Autodesk Fusion 360 part; units mm, degrees
(part 6 of 11)
  spline S88 degree 5 poles (-19.33, -28.8285) (-19.3279, -28.8303) (-19.3238, -28.8339) (-19.3174, -28.8391) (-19.3087, -28.8458) (-19.2974, -28.8537) (-19.286, -28.8614) (-19.2743, -28.8689) (-19.2626, -28.8762) (-19.2508, -28.8835) (-19.2389, -28.8907) (-19.227, -28.8979) (-19.215, -28.9049) (-19.2028, -28.9117) (-19.1905, -28.9185) (-19.1782, -28.925) (-19.1657, -28.9315) (-19.1531, -28.9379) (-19.1405, -28.9442) (-19.1278, -28.9504) (-19.1151, -28.9565) (-19.1022, -28.9625) (-19.0894, -28.9684) (-19.0764, -28.9743) (-19.0634, -28.98) (-19.0503, -28.9857) (-19.0371, -28.9913) (-19.0239, -28.9968) (-19.0106, -29.0022) (-18.9972, -29.0075) (-18.9838, -29.0128) (-18.9704, -29.0179) (-18.9569, -29.0231) (-18.9433, -29.0281) (-18.9297, -29.033) (-18.916, -29.0379) (-18.9023, -29.0427) (-18.8885, -29.0474) (-18.8746, -29.0521) (-18.8608, -29.0566) (-18.8468, -29.0612) (-18.8328, -29.0656) (-18.8188, -29.07) (-18.8047, -29.0742) (-18.7906, -29.0785) (-18.7764, -29.0826) (-18.7622, -29.0867) (-18.7479, -29.0907) (-18.7336, -29.0947) (-18.7193, -29.0985) (-18.7049, -29.1024) (-18.6905, -29.1061) (-18.676, -29.1098) (-18.6614, -29.1134) (-18.6469, -29.1169) (-18.6323, -29.1204) (-18.6176, -29.1238) (-18.6029, -29.1272) (-18.5882, -29.1304) (-18.5734, -29.1337) (-18.5586, -29.1368) (-18.5438, -29.1399) (-18.5289, -29.1429) (-18.514, -29.1459) (-18.499, -29.1488) (-18.484, -29.1516) (-18.469, -29.1544) (-18.4539, -29.1571) (-18.4388, -29.1597) (-18.4237, -29.1623) (-18.4085, -29.1648) (-18.3964, -29.1667) (-18.3872, -29.1682) (-18.3811, -29.1691) (-18.3781, -29.1696) knots 0 0 0 0 0 0 0.01428571 0.02857143 0.04285714 0.05714286 0.07142857 0.08571429 0.1 0.11428571 0.12857143 0.14285714 0.15714286 0.17142857 0.18571429 0.2 0.21428571 0.22857143 0.24285714 0.25714286 0.27142857 0.28571429 0.3 0.31428571 0.32857143 0.34285714 0.35714286 0.37142857 0.38571429 0.4 0.41428571 0.42857143 0.44285714 0.45714286 0.47142857 0.48571429 0.5 0.51428571 0.52857143 0.54285714 0.55714286 0.57142857 0.58571429 0.6 0.61428571 0.62857143 0.64285714 0.65714286 0.67142857 0.68571429 0.7 0.71428571 0.72857143 0.74285714 0.75714286 0.77142857 0.78571429 0.8 0.81428571 0.82857143 0.84285714 0.85714286 0.87142857 0.88571429 0.9 0.91428571 0.92857143 0.94285714 0.95714286 0.97142857 0.98571429 1 1 1 1 1 1 construction
  arc A179 (-18.3781, -29.1696) -> (-18.141, -28.8555) centre (-23.9648, -24.7074) ccw construction
  spline S89 degree 5 poles (-18.141, -28.8555) (-18.1423, -28.8527) (-18.1449, -28.8471) (-18.1488, -28.8387) (-18.154, -28.8275) (-18.1606, -28.8136) (-18.1672, -28.7998) (-18.1739, -28.786) (-18.1807, -28.7722) (-18.1874, -28.7585) (-18.1943, -28.7449) (-18.2012, -28.7313) (-18.2081, -28.7178) (-18.2151, -28.7043) (-18.2221, -28.6909) (-18.2292, -28.6775) (-18.2364, -28.6642) (-18.2435, -28.6509) (-18.2508, -28.6377) (-18.2581, -28.6245) (-18.2654, -28.6114) (-18.2728, -28.5984) (-18.2803, -28.5854) (-18.2878, -28.5725) (-18.2954, -28.5597) (-18.303, -28.5469) (-18.3107, -28.5341) (-18.3184, -28.5214) (-18.3261, -28.5088) (-18.334, -28.4963) (-18.3419, -28.4838) (-18.3498, -28.4714) (-18.3578, -28.459) (-18.3658, -28.4467) (-18.3739, -28.4345) (-18.3821, -28.4223) (-18.3903, -28.4102) (-18.3986, -28.3982) (-18.4069, -28.3862) (-18.4153, -28.3743) (-18.4237, -28.3625) (-18.4322, -28.3508) (-18.4408, -28.3391) (-18.4494, -28.3275) (-18.4581, -28.316) (-18.4668, -28.3046) (-18.4756, -28.2932) (-18.4844, -28.2819) (-18.4933, -28.2707) (-18.5023, -28.2595) (-18.5114, -28.2485) (-18.5205, -28.2376) (-18.5296, -28.2267) (-18.5389, -28.2159) (-18.5482, -28.2053) (-18.5576, -28.1947) (-18.567, -28.1842) (-18.5765, -28.1737) (-18.5861, -28.1634) (-18.5957, -28.1532) (-18.6054, -28.1431) (-18.6153, -28.1332) (-18.6252, -28.1234) (-18.6353, -28.1137) (-18.6454, -28.1042) (-18.6556, -28.0947) (-18.6658, -28.0854) (-18.6761, -28.0761) (-18.6865, -28.067) (-18.697, -28.0581) (-18.7077, -28.0494) (-18.7166, -28.0429) (-18.7233, -28.0382) (-18.7279, -28.0352) (-18.7303, -28.0337) knots -1 -1 -1 -1 -1 -1 -0.98571429 -0.97142857 -0.95714286 -0.94285714 -0.92857143 -0.91428571 -0.9 -0.88571429 -0.87142857 -0.85714286 -0.84285714 -0.82857143 -0.81428571 -0.8 -0.78571429 -0.77142857 -0.75714286 -0.74285714 -0.72857143 -0.71428571 -0.7 -0.68571429 -0.67142857 -0.65714286 -0.64285714 -0.62857143 -0.61428571 -0.6 -0.58571429 -0.57142857 -0.55714286 -0.54285714 -0.52857143 -0.51428571 -0.5 -0.48571429 -0.47142857 -0.45714286 -0.44285714 -0.42857143 -0.41428571 -0.4 -0.38571429 -0.37142857 -0.35714286 -0.34285714 -0.32857143 -0.31428571 -0.3 -0.28571429 -0.27142857 -0.25714286 -0.24285714 -0.22857143 -0.21428571 -0.2 -0.18571429 -0.17142857 -0.15714286 -0.14285714 -0.12857143 -0.11428571 -0.1 -0.08571429 -0.07142857 -0.05714286 -0.04285714 -0.02857143 -0.01428571 0 0 0 0 0 0 construction
  line L95 (-18.7303, -28.0337) -> (-18.788, -27.9968) construction
  arc A180 (-18.8697, -27.6608) -> (-18.788, -27.9968) centre (-18.6534, -27.7862) ccw construction
  arc A181 (-18.8697, -27.6608) -> (-18.8128, -27.5605) centre (-23.9648, -24.7074) ccw construction
  arc A182 (-18.4826, -27.4579) -> (-18.8128, -27.5605) centre (-18.5941, -27.6816) ccw construction
  line L96 (-18.4826, -27.4579) -> (-18.4213, -27.4885) construction
  spline S90 degree 5 poles (-18.4213, -27.4885) (-18.4188, -27.4897) (-18.4139, -27.4921) (-18.4064, -27.4955) (-18.3962, -27.4997) (-18.3833, -27.5045) (-18.3703, -27.5089) (-18.3571, -27.5131) (-18.3438, -27.5172) (-18.3306, -27.5211) (-18.3172, -27.5251) (-18.3039, -27.5288) (-18.2904, -27.5325) (-18.2769, -27.536) (-18.2633, -27.5393) (-18.2496, -27.5425) (-18.2359, -27.5455) (-18.2221, -27.5484) (-18.2083, -27.5512) (-18.1945, -27.5539) (-18.1806, -27.5565) (-18.1666, -27.559) (-18.1526, -27.5614) (-18.1386, -27.5637) (-18.1245, -27.5659) (-18.1104, -27.5679) (-18.0963, -27.5699) (-18.0821, -27.5718) (-18.0678, -27.5736) (-18.0536, -27.5753) (-18.0392, -27.5769) (-18.0249, -27.5784) (-18.0105, -27.5799) (-17.9961, -27.5812) (-17.9817, -27.5825) (-17.9672, -27.5836) (-17.9527, -27.5847) (-17.9382, -27.5857) (-17.9236, -27.5866) (-17.909, -27.5874) (-17.8944, -27.5882) (-17.8797, -27.5888) (-17.865, -27.5894) (-17.8503, -27.5899) (-17.8356, -27.5904) (-17.8208, -27.5907) (-17.806, -27.591) (-17.7912, -27.5912) (-17.7764, -27.5913) (-17.7615, -27.5913) (-17.7466, -27.5912) (-17.7317, -27.5911) (-17.7168, -27.5909) (-17.7018, -27.5907) (-17.6868, -27.5903) (-17.6718, -27.5899) (-17.6568, -27.5894) (-17.6417, -27.5888) (-17.6266, -27.5882) (-17.6115, -27.5875) (-17.5964, -27.5867) (-17.5813, -27.5858) (-17.5661, -27.5849) (-17.551, -27.5839) (-17.5358, -27.5828) (-17.5205, -27.5816) (-17.5053, -27.5804) (-17.4901, -27.5791) (-17.4748, -27.5778) (-17.4595, -27.5763) (-17.4442, -27.5748) (-17.4319, -27.5736) (-17.4227, -27.5726) (-17.4166, -27.5719) (-17.4135, -27.5716) knots 0 0 0 0 0 0 0.01428571 0.02857143 0.04285714 0.05714286 0.07142857 0.08571429 0.1 0.11428571 0.12857143 0.14285714 0.15714286 0.17142857 0.18571429 0.2 0.21428571 0.22857143 0.24285714 0.25714286 0.27142857 0.28571429 0.3 0.31428571 0.32857143 0.34285714 0.35714286 0.37142857 0.38571429 0.4 0.41428571 0.42857143 0.44285714 0.45714286 0.47142857 0.48571429 0.5 0.51428571 0.52857143 0.54285714 0.55714286 0.57142857 0.58571429 0.6 0.61428571 0.62857143 0.64285714 0.65714286 0.67142857 0.68571429 0.7 0.71428571 0.72857143 0.74285714 0.75714286 0.77142857 0.78571429 0.8 0.81428571 0.82857143 0.84285714 0.85714286 0.87142857 0.88571429 0.9 0.91428571 0.92857143 0.94285714 0.95714286 0.97142857 0.98571429 1 1 1 1 1 1 construction
  arc A183 (-17.4135, -27.5716) -> (-17.2659, -27.2069) centre (-23.9648, -24.7074) ccw construction
  spline S91 degree 5 poles (-17.2659, -27.2069) (-17.2678, -27.2045) (-17.2718, -27.1997) (-17.2777, -27.1926) (-17.2857, -27.1832) (-17.2956, -27.1715) (-17.3056, -27.1598) (-17.3156, -27.1482) (-17.3257, -27.1367) (-17.3358, -27.1252) (-17.3459, -27.1138) (-17.3561, -27.1025) (-17.3663, -27.0912) (-17.3765, -27.08) (-17.3868, -27.0688) (-17.3971, -27.0577) (-17.4075, -27.0467) (-17.4178, -27.0358) (-17.4283, -27.0249) (-17.4387, -27.0141) (-17.4492, -27.0033) (-17.4597, -26.9927) (-17.4703, -26.982) (-17.4809, -26.9715) (-17.4915, -26.9611) (-17.5022, -26.9507) (-17.5129, -26.9403) (-17.5236, -26.9301) (-17.5344, -26.9199) (-17.5452, -26.9098) (-17.5561, -26.8998) (-17.5669, -26.8898) (-17.5779, -26.88) (-17.5888, -26.8702) (-17.5998, -26.8605) (-17.6108, -26.8508) (-17.6219, -26.8413) (-17.633, -26.8318) (-17.6441, -26.8224) (-17.6553, -26.8131) (-17.6665, -26.8038) (-17.6778, -26.7947) (-17.689, -26.7856) (-17.7004, -26.7767) (-17.7117, -26.7678) (-17.7231, -26.759) (-17.7345, -26.7503) (-17.746, -26.7417) (-17.7575, -26.7332) (-17.7691, -26.7247) (-17.7807, -26.7164) (-17.7923, -26.7082) (-17.804, -26.7001) (-17.8157, -26.6921) (-17.8274, -26.6842) (-17.8392, -26.6764) (-17.8511, -26.6687) (-17.863, -26.6611) (-17.8749, -26.6536) (-17.8868, -26.6462) (-17.8988, -26.6389) (-17.9109, -26.6319) (-17.923, -26.625) (-17.9352, -26.6183) (-17.9475, -26.6117) (-17.9598, -26.6052) (-17.9721, -26.5988) (-17.9844, -26.5926) (-17.9968, -26.5864) (-18.0093, -26.5805) (-18.0219, -26.5749) (-18.0321, -26.5709) (-18.0399, -26.5681) (-18.0451, -26.5664) (-18.0477, -26.5656) knots -1 -1 -1 -1 -1 -1 -0.98571429 -0.97142857 -0.95714286 -0.94285714 -0.92857143 -0.91428571 -0.9 -0.88571429 -0.87142857 -0.85714286 -0.84285714 -0.82857143 -0.81428571 -0.8 -0.78571429 -0.77142857 -0.75714286 -0.74285714 -0.72857143 -0.71428571 -0.7 -0.68571429 -0.67142857 -0.65714286 -0.64285714 -0.62857143 -0.61428571 -0.6 -0.58571429 -0.57142857 -0.55714286 -0.54285714 -0.52857143 -0.51428571 -0.5 -0.48571429 -0.47142857 -0.45714286 -0.44285714 -0.42857143 -0.41428571 -0.4 -0.38571429 -0.37142857 -0.35714286 -0.34285714 -0.32857143 -0.31428571 -0.3 -0.28571429 -0.27142857 -0.25714286 -0.24285714 -0.22857143 -0.21428571 -0.2 -0.18571429 -0.17142857 -0.15714286 -0.14285714 -0.12857143 -0.11428571 -0.1 -0.08571429 -0.07142857 -0.05714286 -0.04285714 -0.02857143 -0.01428571 0 0 0 0 0 0 construction
  line L97 (-18.0477, -26.5656) -> (-18.113, -26.5449) construction
  arc A184 (-18.2789, -26.2414) -> (-18.113, -26.5449) centre (-18.0375, -26.3066) ccw construction
  arc A185 (-18.2789, -26.2414) -> (-18.2499, -26.1299) centre (-23.9648, -24.7074) ccw construction
  arc A186 (-17.9575, -25.9453) -> (-18.2499, -26.1299) centre (-18.0073, -26.1903) ccw construction
  line L98 (-17.9575, -25.9453) -> (-17.8904, -25.9589) construction
  spline S92 degree 5 poles (-17.8904, -25.9589) (-17.8877, -25.9595) (-17.8823, -25.9605) (-17.8742, -25.9619) (-17.8633, -25.9633) (-17.8496, -25.9646) (-17.8358, -25.9655) (-17.822, -25.9661) (-17.8082, -25.9666) (-17.7943, -25.967) (-17.7804, -25.9674) (-17.7665, -25.9676) (-17.7526, -25.9676) (-17.7386, -25.9675) (-17.7246, -25.9672) (-17.7106, -25.9667) (-17.6966, -25.966) (-17.6825, -25.9653) (-17.6685, -25.9644) (-17.6544, -25.9634) (-17.6403, -25.9623) (-17.6261, -25.9612) (-17.612, -25.9599) (-17.5979, -25.9584) (-17.5837, -25.9569) (-17.5695, -25.9553) (-17.5553, -25.9535) (-17.5411, -25.9516) (-17.5269, -25.9497) (-17.5127, -25.9476) (-17.4985, -25.9455) (-17.4842, -25.9433) (-17.47, -25.9409) (-17.4557, -25.9385) (-17.4414, -25.936) (-17.4272, -25.9333) (-17.4129, -25.9306) (-17.3986, -25.9278) (-17.3843, -25.9249) (-17.3699, -25.922) (-17.3556, -25.9189) (-17.3413, -25.9157) (-17.327, -25.9125) (-17.3126, -25.9092) (-17.2983, -25.9058) (-17.2839, -25.9023) (-17.2696, -25.8987) (-17.2552, -25.8951) (-17.2408, -25.8913) (-17.2265, -25.8875) (-17.2121, -25.8836) (-17.1977, -25.8796) (-17.1833, -25.8756) (-17.169, -25.8714) (-17.1546, -25.8672) (-17.1402, -25.8629) (-17.1258, -25.8586) (-17.1114, -25.8541) (-17.097, -25.8496) (-17.0826, -25.845) (-17.0682, -25.8403) (-17.0538, -25.8356) (-17.0394, -25.8307) (-17.025, -25.8258) (-17.0106, -25.8209) (-16.9962, -25.8158) (-16.9818, -25.8107) (-16.9674, -25.8055) (-16.953, -25.8002) (-16.9386, -25.7949) (-16.9242, -25.7895) (-16.9127, -25.7851) (-16.9041, -25.7818) (-16.8983, -25.7795) (-16.8954, -25.7784) knots 0 0 0 0 0 0 0.01428571 0.02857143 0.04285714 0.05714286 0.07142857 0.08571429 0.1 0.11428571 0.12857143 0.14285714 0.15714286 0.17142857 0.18571429 0.2 0.21428571 0.22857143 0.24285714 0.25714286 0.27142857 0.28571429 0.3 0.31428571 0.32857143 0.34285714 0.35714286 0.37142857 0.38571429 0.4 0.41428571 0.42857143 0.44285714 0.45714286 0.47142857 0.48571429 0.5 0.51428571 0.52857143 0.54285714 0.55714286 0.57142857 0.58571429 0.6 0.61428571 0.62857143 0.64285714 0.65714286 0.67142857 0.68571429 0.7 0.71428571 0.72857143 0.74285714 0.75714286 0.77142857 0.78571429 0.8 0.81428571 0.82857143 0.84285714 0.85714286 0.87142857 0.88571429 0.9 0.91428571 0.92857143 0.94285714 0.95714286 0.97142857 0.98571429 1 1 1 1 1 1 construction
  arc A187 (-16.8954, -25.7784) -> (-16.8472, -25.3879) centre (-23.9648, -24.7074) ccw construction
  spline S93 degree 5 poles (-16.8472, -25.3879) (-16.8497, -25.3861) (-16.8548, -25.3825) (-16.8624, -25.3772) (-16.8725, -25.3702) (-16.8851, -25.3614) (-16.8978, -25.3527) (-16.9105, -25.3441) (-16.9232, -25.3356) (-16.9359, -25.3271) (-16.9486, -25.3187) (-16.9614, -25.3104) (-16.9742, -25.3021) (-16.9869, -25.294) (-16.9998, -25.2858) (-17.0126, -25.2778) (-17.0254, -25.2698) (-17.0383, -25.262) (-17.0512, -25.2541) (-17.0641, -25.2464) (-17.077, -25.2387) (-17.0899, -25.2312) (-17.1029, -25.2236) (-17.1158, -25.2162) (-17.1288, -25.2089) (-17.1418, -25.2016) (-17.1548, -25.1944) (-17.1678, -25.1873) (-17.1809, -25.1802) (-17.1939, -25.1733) (-17.207, -25.1664) (-17.2201, -25.1596) (-17.2332, -25.1529) (-17.2463, -25.1463) (-17.2594, -25.1397) (-17.2726, -25.1333) (-17.2857, -25.1269) (-17.2989, -25.1206) (-17.3121, -25.1144) (-17.3253, -25.1083) (-17.3385, -25.1023) (-17.3517, -25.0964) (-17.365, -25.0906) (-17.3782, -25.0848) (-17.3915, -25.0792) (-17.4048, -25.0736) (-17.4181, -25.0682) (-17.4314, -25.0628) (-17.4447, -25.0576) (-17.4581, -25.0524) (-17.4714, -25.0474) (-17.4848, -25.0424) (-17.4982, -25.0376) (-17.5115, -25.0329) (-17.525, -25.0283) (-17.5384, -25.0239) (-17.5518, -25.0195) (-17.5652, -25.0152) (-17.5787, -25.0111) (-17.5921, -25.007) (-17.6056, -25.0032) (-17.6191, -24.9994) (-17.6326, -24.9959) (-17.6461, -24.9926) (-17.6597, -24.9894) (-17.6732, -24.9863) (-17.6868, -24.9834) (-17.7003, -24.9805) (-17.7139, -24.9778) (-17.7274, -24.9753) (-17.741, -24.9732) (-17.7519, -24.9719) (-17.7602, -24.9712) (-17.7656, -24.9709) (-17.7684, -24.9708) knots -1 -1 -1 -1 -1 -1 -0.98571429 -0.97142857 -0.95714286 -0.94285714 -0.92857143 -0.91428571 -0.9 -0.88571429 -0.87142857 -0.85714286 -0.84285714 -0.82857143 -0.81428571 -0.8 -0.78571429 -0.77142857 -0.75714286 -0.74285714 -0.72857143 -0.71428571 -0.7 -0.68571429 -0.67142857 -0.65714286 -0.64285714 -0.62857143 -0.61428571 -0.6 -0.58571429 -0.57142857 -0.55714286 -0.54285714 -0.52857143 -0.51428571 -0.5 -0.48571429 -0.47142857 -0.45714286 -0.44285714 -0.42857143 -0.41428571 -0.4 -0.38571429 -0.37142857 -0.35714286 -0.34285714 -0.32857143 -0.31428571 -0.3 -0.28571429 -0.27142857 -0.25714286 -0.24285714 -0.22857143 -0.21428571 -0.2 -0.18571429 -0.17142857 -0.15714286 -0.14285714 -0.12857143 -0.11428571 -0.1 -0.08571429 -0.07142857 -0.05714286 -0.04285714 -0.02857143 -0.01428571 0 0 0 0 0 0 construction
  line L99 (-17.7684, -24.9708) -> (-17.8368, -24.9677) construction
  arc A188 (-18.0756, -24.7176) -> (-17.8368, -24.9677) centre (-17.8256, -24.718) ccw construction
  arc A189 (-18.0756, -24.7176) -> (-18.0765, -24.6023) centre (-23.9648, -24.7074) ccw construction
  arc A190 (-17.8418, -24.3483) -> (-18.0765, -24.6023) centre (-17.8265, -24.5979) ccw construction
  line L100 (-17.8418, -24.3483) -> (-17.7734, -24.3441) construction
  spline S94 degree 5 poles (-17.7734, -24.3441) (-17.7707, -24.344) (-17.7652, -24.3436) (-17.757, -24.3428) (-17.7461, -24.3413) (-17.7326, -24.339) (-17.719, -24.3363) (-17.7055, -24.3333) (-17.692, -24.3303) (-17.6785, -24.3271) (-17.665, -24.3238) (-17.6515, -24.3204) (-17.6381, -24.3168) (-17.6246, -24.3131) (-17.6112, -24.3092) (-17.5978, -24.3051) (-17.5844, -24.3008) (-17.571, -24.2965) (-17.5577, -24.292) (-17.5443, -24.2874) (-17.531, -24.2827) (-17.5176, -24.2779) (-17.5043, -24.273) (-17.491, -24.2679) (-17.4777, -24.2628) (-17.4645, -24.2575) (-17.4512, -24.2522) (-17.438, -24.2467) (-17.4248, -24.2411) (-17.4116, -24.2355) (-17.3984, -24.2297) (-17.3852, -24.2239) (-17.372, -24.2179) (-17.3589, -24.2119) (-17.3457, -24.2057) (-17.3326, -24.1995) (-17.3195, -24.1932) (-17.3064, -24.1868) (-17.2934, -24.1803) (-17.2803, -24.1737) (-17.2673, -24.167) (-17.2542, -24.1603) (-17.2412, -24.1534) (-17.2282, -24.1465) (-17.2153, -24.1395) (-17.2023, -24.1324) (-17.1894, -24.1253) (-17.1764, -24.118) (-17.1635, -24.1107) (-17.1506, -24.1033) (-17.1378, -24.0958) (-17.1249, -24.0882) (-17.1121, -24.0806) (-17.0992, -24.0729) (-17.0864, -24.0651) (-17.0737, -24.0572) (-17.0609, -24.0493) (-17.0481, -24.0413) (-17.0354, -24.0332) (-17.0227, -24.025) (-17.01, -24.0168) (-16.9973, -24.0084) (-16.9847, -24) (-16.972, -23.9916) (-16.9594, -23.9831) (-16.9468, -23.9745) (-16.9342, -23.9658) (-16.9216, -23.957) (-16.9091, -23.9482) (-16.8966, -23.9393) (-16.8841, -23.9304) (-16.8741, -23.9232) (-16.8666, -23.9177) (-16.8616, -23.9141) (-16.8591, -23.9123) knots 0 0 0 0 0 0 0.01428571 0.02857143 0.04285714 0.05714286 0.07142857 0.08571429 0.1 0.11428571 0.12857143 0.14285714 0.15714286 0.17142857 0.18571429 0.2 0.21428571 0.22857143 0.24285714 0.25714286 0.27142857 0.28571429 0.3 0.31428571 0.32857143 0.34285714 0.35714286 0.37142857 0.38571429 0.4 0.41428571 0.42857143 0.44285714 0.45714286 0.47142857 0.48571429 0.5 0.51428571 0.52857143 0.54285714 0.55714286 0.57142857 0.58571429 0.6 0.61428571 0.62857143 0.64285714 0.65714286 0.67142857 0.68571429 0.7 0.71428571 0.72857143 0.74285714 0.75714286 0.77142857 0.78571429 0.8 0.81428571 0.82857143 0.84285714 0.85714286 0.87142857 0.88571429 0.9 0.91428571 0.92857143 0.94285714 0.95714286 0.97142857 0.98571429 1 1 1 1 1 1 construction
  arc A191 (-16.8591, -23.9123) -> (-16.9136, -23.5225) centre (-23.9648, -24.7074) ccw construction
  spline S95 degree 5 poles (-16.9136, -23.5225) (-16.9165, -23.5215) (-16.9223, -23.5193) (-16.931, -23.5162) (-16.9426, -23.512) (-16.9571, -23.5068) (-16.9715, -23.5017) (-16.986, -23.4966) (-17.0005, -23.4917) (-17.015, -23.4868) (-17.0295, -23.482) (-17.0439, -23.4772) (-17.0584, -23.4726) (-17.0729, -23.468) (-17.0874, -23.4635) (-17.1018, -23.459) (-17.1163, -23.4546) (-17.1308, -23.4504) (-17.1452, -23.4461) (-17.1597, -23.442) (-17.1742, -23.4379) (-17.1886, -23.434) (-17.2031, -23.4301) (-17.2175, -23.4262) (-17.2319, -23.4225) (-17.2464, -23.4188) (-17.2608, -23.4152) (-17.2752, -23.4117) (-17.2896, -23.4083) (-17.3041, -23.405) (-17.3185, -23.4017) (-17.3329, -23.3985) (-17.3472, -23.3955) (-17.3616, -23.3924) (-17.376, -23.3895) (-17.3904, -23.3867) (-17.4047, -23.3839) (-17.4191, -23.3813) (-17.4334, -23.3787) (-17.4478, -23.3762) (-17.4621, -23.3738) (-17.4764, -23.3715) (-17.4907, -23.3693) (-17.505, -23.3672) (-17.5193, -23.3652) (-17.5335, -23.3633) (-17.5478, -23.3615) (-17.562, -23.3598) (-17.5763, -23.3581) (-17.5905, -23.3566) (-17.6047, -23.3552) (-17.6189, -23.3539) (-17.633, -23.3527) (-17.6472, -23.3516) (-17.6613, -23.3507) (-17.6754, -23.3498) (-17.6895, -23.3491) (-17.7036, -23.3484) (-17.7177, -23.3479) (-17.7317, -23.3475) (-17.7457, -23.3472) (-17.7597, -23.3471) (-17.7737, -23.3472) (-17.7876, -23.3475) (-17.8015, -23.3479) (-17.8154, -23.3485) (-17.8292, -23.3491) (-17.8431, -23.3498) (-17.8569, -23.3507) (-17.8706, -23.3518) (-17.8843, -23.3533) (-17.8952, -23.3549) (-17.9033, -23.3564) (-17.9087, -23.3575) (-17.9114, -23.3581) knots -1 -1 -1 -1 -1 -1 -0.98571429 -0.97142857 -0.95714286 -0.94285714 -0.92857143 -0.91428571 -0.9 -0.88571429 -0.87142857 -0.85714286 -0.84285714 -0.82857143 -0.81428571 -0.8 -0.78571429 -0.77142857 -0.75714286 -0.74285714 -0.72857143 -0.71428571 -0.7 -0.68571429 -0.67142857 -0.65714286 -0.64285714 -0.62857143 -0.61428571 -0.6 -0.58571429 -0.57142857 -0.55714286 -0.54285714 -0.52857143 -0.51428571 -0.5 -0.48571429 -0.47142857 -0.45714286 -0.44285714 -0.42857143 -0.41428571 -0.4 -0.38571429 -0.37142857 -0.35714286 -0.34285714 -0.32857143 -0.31428571 -0.3 -0.28571429 -0.27142857 -0.25714286 -0.24285714 -0.22857143 -0.21428571 -0.2 -0.18571429 -0.17142857 -0.15714286 -0.14285714 -0.12857143 -0.11428571 -0.1 -0.08571429 -0.07142857 -0.05714286 -0.04285714 -0.02857143 -0.01428571 0 0 0 0 0 0 construction
  line L101 (-17.9114, -23.3581) -> (-17.9782, -23.3728) construction
  arc A192 (-18.2736, -23.193) -> (-17.9782, -23.3728) centre (-18.032, -23.1287) ccw construction
  circle A193 centre (-23.9648, -24.7074) radius 1.25 construction
  circle A194 centre (-23.9648, -24.7074) radius 1.225 construction
  circle A195 centre (-11.6741, -19.5) radius 1.225 construction
  line L102 (-7.5589, -33.5042) -> (-9.5095, -28.9004) construction
  line L103 (-9.5095, -28.9004) -> (-5.8324, -16.7546) construction
  arc A196 (-5.8324, -16.7546) -> (-7.9044, -14.1813) centre (-7.7466, -16.1751) ccw construction
  line L104 (-7.9044, -14.1813) -> (-14.4255, -14.1704) construction
  arc A197 (-14.4255, -14.1704) -> (-16.9722, -14.6854) centre (-14.4364, -20.6704) ccw construction
  line L105 (-16.9722, -14.6854) -> (-23.7382, -17.5521) construction
  arc A198 (-23.7382, -17.5521) -> (-25.8797, -19.0234) centre (-21.2025, -23.537) ccw construction
  line L106 (-25.8797, -19.0234) -> (-30.4081, -23.7158) construction
  arc A199 (-30.4081, -23.7158) -> (-30.0007, -26.9945) centre (-29.0855, -25.2161) ccw construction
  line L107 (-30.0007, -26.9945) -> (-18.7172, -32.8016) construction
  line L108 (-18.7172, -32.8016) -> (-16.7666, -37.4054) construction
  line L109 (-16.7666, -37.4054) -> (-7.5589, -33.5042) construction
  line L110 (-20.3552, -16.1187) -> (-12.1627, -35.4548) construction
  line L111 (-32.6369, -35.6954) -> (-24.2895, -27.0745)
  line L112 (-24.2895, -27.0745) -> (-25.7264, -25.6832)
  line L113 (-25.7264, -25.6832) -> (-34.0738, -34.3042)
  line L114 (-34.0738, -34.3042) -> (-32.6369, -35.6954)
  point P0 (-3.7477, -19.9132)
  dimension "d196" = 12
  dimension "d197" = 2
  constraint horizontal L48
  constraint perpendicular L48 L49
  constraint parallel L48 L50
  constraint parallel L49 L51
  constraint coincident L52 P0
  constraint coincident L53 P0
  constraint midpoint L105 L110.start
  constraint midpoint L109 L110.end
  constraint symmetric L48.start L110 L111.start
  constraint symmetric L48.end L110 L111.end
  constraint symmetric L49.end L110 L112.end
  constraint symmetric L50.end L110 L113.end
  measures "d196" distance of L49.end L50.end
  measures "d197" distance of L48.end L49.end
extrude "Extrude1''" add sketch "Sketch21" along normal blind 2 separate body contours A89 L44 S44 A90 S45 L45 A91 A92 A93 L46 S46 L48 L50 L51 | A89 L44 S44 A90 S45 L45 A91 A92 A93 L46 S46 L48 L49 L50 makes body 4 in component "Component"
sketch "Sketch22" plane through (0, 0, 5.45) normal (0, 0, 1) x (-1, 0, 0)
  arc A0 (-17.5052, -18.6742) -> (-17.5202, -18.7885) centre (-11.6741, -19.5) ccw
  arc A1 (-17.7878, -19.0075) -> (-17.5202, -18.7885) centre (-17.7684, -18.7583) ccw
  line L0 (-17.7878, -19.0075) -> (-17.8561, -19.0022)
  spline S0 degree 5 poles (-17.8561, -19.0022) (-17.8588, -19.002) (-17.8643, -19.0016) (-17.8726, -19.0013) (-17.8835, -19.0012) (-17.8973, -19.0016) (-17.9111, -19.0024) (-17.9249, -19.0035) (-17.9387, -19.0046) (-17.9525, -19.0059) (-17.9663, -19.0073) (-17.9801, -19.0088) (-17.9939, -19.0105) (-18.0078, -19.0123) (-18.0216, -19.0143) (-18.0355, -19.0165) (-18.0493, -19.0189) (-18.0632, -19.0214) (-18.077, -19.024) (-18.0909, -19.0267) (-18.1048, -19.0295) (-18.1186, -19.0324) (-18.1325, -19.0354) (-18.1463, -19.0385) (-18.1602, -19.0418) (-18.1741, -19.0452) (-18.188, -19.0486) (-18.2018, -19.0522) (-18.2157, -19.0559) (-18.2295, -19.0597) (-18.2434, -19.0636) (-18.2573, -19.0675) (-18.2711, -19.0716) (-18.285, -19.0758) (-18.2989, -19.08) (-18.3127, -19.0844) (-18.3266, -19.0888) (-18.3404, -19.0933) (-18.3542, -19.098) (-18.3681, -19.1027) (-18.3819, -19.1075) (-18.3958, -19.1123) (-18.4096, -19.1173) (-18.4234, -19.1224) (-18.4372, -19.1275) (-18.4511, -19.1327) (-18.4649, -19.138) (-18.4787, -19.1434) (-18.4925, -19.1489) (-18.5063, -19.1544) (-18.52, -19.1601) (-18.5338, -19.1658) (-18.5476, -19.1716) (-18.5614, -19.1774) (-18.5751, -19.1834) (-18.5889, -19.1894) (-18.6026, -19.1955) (-18.6164, -19.2017) (-18.6301, -19.2079) (-18.6438, -19.2143) (-18.6575, -19.2207) (-18.6712, -19.2271) (-18.6849, -19.2337) (-18.6986, -19.2403) (-18.7123, -19.247) (-18.726, -19.2538) (-18.7397, -19.2606) (-18.7533, -19.2676) (-18.767, -19.2746) (-18.7806, -19.2816) (-18.7942, -19.2887) (-18.8051, -19.2945) (-18.8133, -19.2989) (-18.8187, -19.3018) (-18.8214, -19.3032) knots 0 0 0 0 0 0 0.01428571 0.02857143 0.04285714 0.05714286 0.07142857 0.08571429 0.1 0.11428571 0.12857143 0.14285714 0.15714286 0.17142857 0.18571429 0.2 0.21428571 0.22857143 0.24285714 0.25714286 0.27142857 0.28571429 0.3 0.31428571 0.32857143 0.34285714 0.35714286 0.37142857 0.38571429 0.4 0.41428571 0.42857143 0.44285714 0.45714286 0.47142857 0.48571429 0.5 0.51428571 0.52857143 0.54285714 0.55714286 0.57142857 0.58571429 0.6 0.61428571 0.62857143 0.64285714 0.65714286 0.67142857 0.68571429 0.7 0.71428571 0.72857143 0.74285714 0.75714286 0.77142857 0.78571429 0.8 0.81428571 0.82857143 0.84285714 0.85714286 0.87142857 0.88571429 0.9 0.91428571 0.92857143 0.94285714 0.95714286 0.97142857 0.98571429 1 1 1 1 1 1
  arc A2 (-18.8214, -19.3032) -> (-18.8214, -19.6968) centre (-11.6741, -19.5) ccw
  spline S1 degree 5 poles (-18.8214, -19.6968) (-18.8187, -19.6982) (-18.8133, -19.7011) (-18.8051, -19.7055) (-18.7942, -19.7113) (-18.7806, -19.7184) (-18.767, -19.7254) (-18.7533, -19.7324) (-18.7397, -19.7394) (-18.726, -19.7462) (-18.7123, -19.753) (-18.6986, -19.7597) (-18.6849, -19.7663) (-18.6712, -19.7729) (-18.6575, -19.7793) (-18.6438, -19.7857) (-18.6301, -19.7921) (-18.6164, -19.7983) (-18.6026, -19.8045) (-18.5889, -19.8106) (-18.5751, -19.8166) (-18.5614, -19.8226) (-18.5476, -19.8284) (-18.5338, -19.8342) (-18.52, -19.8399) (-18.5063, -19.8456) (-18.4925, -19.8511) (-18.4787, -19.8566) (-18.4649, -19.862) (-18.4511, -19.8673) (-18.4372, -19.8725) (-18.4234, -19.8776) (-18.4096, -19.8827) (-18.3958, -19.8877) (-18.3819, -19.8925) (-18.3681, -19.8973) (-18.3542, -19.902) (-18.3404, -19.9067) (-18.3266, -19.9112) (-18.3127, -19.9156) (-18.2989, -19.92) (-18.285, -19.9242) (-18.2711, -19.9284) (-18.2573, -19.9325) (-18.2434, -19.9364) (-18.2295, -19.9403) (-18.2157, -19.9441) (-18.2018, -19.9478) (-18.188, -19.9514) (-18.1741, -19.9548) (-18.1602, -19.9582) (-18.1463, -19.9615) (-18.1325, -19.9646) (-18.1186, -19.9676) (-18.1048, -19.9705) (-18.0909, -19.9733) (-18.077, -19.976) (-18.0632, -19.9786) (-18.0493, -19.9811) (-18.0355, -19.9835) (-18.0216, -19.9857) (-18.0078, -19.9877) (-17.9939, -19.9895) (-17.9801, -19.9912) (-17.9663, -19.9927) (-17.9525, -19.9941) (-17.9387, -19.9954) (-17.9249, -19.9965) (-17.9111, -19.9976) (-17.8973, -19.9984) (-17.8835, -19.9988) (-17.8726, -19.9987) (-17.8643, -19.9984) (-17.8588, -19.998) (-17.8561, -19.9978) knots -1 -1 -1 -1 -1 -1 -0.98571429 -0.97142857 -0.95714286 -0.94285714 -0.92857143 -0.91428571 -0.9 -0.88571429 -0.87142857 -0.85714286 -0.84285714 -0.82857143 -0.81428571 -0.8 -0.78571429 -0.77142857 -0.75714286 -0.74285714 -0.72857143 -0.71428571 -0.7 -0.68571429 -0.67142857 -0.65714286 -0.64285714 -0.62857143 -0.61428571 -0.6 -0.58571429 -0.57142857 -0.55714286 -0.54285714 -0.52857143 -0.51428571 -0.5 -0.48571429 -0.47142857 -0.45714286 -0.44285714 -0.42857143 -0.41428571 -0.4 -0.38571429 -0.37142857 -0.35714286 -0.34285714 -0.32857143 -0.31428571 -0.3 -0.28571429 -0.27142857 -0.25714286 -0.24285714 -0.22857143 -0.21428571 -0.2 -0.18571429 -0.17142857 -0.15714286 -0.14285714 -0.12857143 -0.11428571 -0.1 -0.08571429 -0.07142857 -0.05714286 -0.04285714 -0.02857143 -0.01428571 0 0 0 0 0 0
  line L1 (-17.8561, -19.9978) -> (-17.7878, -19.9925)
  arc A3 (-17.5202, -20.2115) -> (-17.7878, -19.9925) centre (-17.7684, -20.2417) ccw
  arc A4 (-17.5202, -20.2115) -> (-17.5052, -20.3258) centre (-11.6741, -19.5) ccw
  arc A5 (-17.707, -20.6066) -> (-17.5052, -20.3258) centre (-17.7527, -20.3608) ccw
  line L2 (-17.707, -20.6066) -> (-17.7743, -20.6192)
  spline S2 degree 5 poles (-17.7743, -20.6192) (-17.777, -20.6197) (-17.7824, -20.6207) (-17.7904, -20.6225) (-17.8011, -20.6253) (-17.8142, -20.6293) (-17.8273, -20.6336) (-17.8404, -20.6382) (-17.8534, -20.6429) (-17.8664, -20.6477) (-17.8794, -20.6526) (-17.8924, -20.6577) (-17.9053, -20.6628) (-17.9182, -20.6682) (-17.931, -20.6737) (-17.9438, -20.6794) (-17.9566, -20.6853) (-17.9694, -20.6913) (-17.9821, -20.6974) (-17.9948, -20.7036) (-18.0074, -20.7099) (-18.0201, -20.7162) (-18.0327, -20.7228) (-18.0453, -20.7294) (-18.0578, -20.7361) (-18.0703, -20.743) (-18.0828, -20.7499) (-18.0953, -20.757) (-18.1077, -20.7641) (-18.1201, -20.7713) (-18.1325, -20.7787) (-18.1449, -20.7861) (-18.1572, -20.7936) (-18.1695, -20.8012) (-18.1818, -20.8089) (-18.1941, -20.8167) (-18.2063, -20.8246) (-18.2185, -20.8325) (-18.2307, -20.8406) (-18.2428, -20.8487) (-18.255, -20.8569) (-18.2671, -20.8652) (-18.2791, -20.8736) (-18.2912, -20.8821) (-18.3032, -20.8906) (-18.3152, -20.8992) (-18.3272, -20.9079) (-18.3391, -20.9167) (-18.351, -20.9256) (-18.3629, -20.9345) (-18.3748, -20.9435) (-18.3866, -20.9526) (-18.3984, -20.9617) (-18.4102, -20.971) (-18.4219, -20.9803) (-18.4337, -20.9896) (-18.4454, -20.9991) (-18.457, -21.0086) (-18.4687, -21.0182) (-18.4803, -21.0279) (-18.4919, -21.0376) (-18.5034, -21.0474) (-18.515, -21.0573) (-18.5265, -21.0672) (-18.538, -21.0773) (-18.5494, -21.0873) (-18.5609, -21.0975) (-18.5723, -21.1077) (-18.5836, -21.118) (-18.595, -21.1283) (-18.6063, -21.1388) (-18.6153, -21.1471) (-18.6221, -21.1535) (-18.6266, -21.1577) (-18.6288, -21.1598) knots 0 0 0 0 0 0 0.01428571 0.02857143 0.04285714 0.05714286 0.07142857 0.08571429 0.1 0.11428571 0.12857143 0.14285714 0.15714286 0.17142857 0.18571429 0.2 0.21428571 0.22857143 0.24285714 0.25714286 0.27142857 0.28571429 0.3 0.31428571 0.32857143 0.34285714 0.35714286 0.37142857 0.38571429 0.4 0.41428571 0.42857143 0.44285714 0.45714286 0.47142857 0.48571429 0.5 0.51428571 0.52857143 0.54285714 0.55714286 0.57142857 0.58571429 0.6 0.61428571 0.62857143 0.64285714 0.65714286 0.67142857 0.68571429 0.7 0.71428571 0.72857143 0.74285714 0.75714286 0.77142857 0.78571429 0.8 0.81428571 0.82857143 0.84285714 0.85714286 0.87142857 0.88571429 0.9 0.91428571 0.92857143 0.94285714 0.95714286 0.97142857 0.98571429 1 1 1 1 1 1
  arc A6 (-18.6288, -21.1598) -> (-18.527, -21.5399) centre (-11.6741, -19.5) ccw
  spline S3 degree 5 poles (-18.527, -21.5399) (-18.524, -21.5406) (-18.518, -21.542) (-18.5089, -21.5441) (-18.4969, -21.5469) (-18.4819, -21.5502) (-18.4669, -21.5535) (-18.4519, -21.5567) (-18.437, -21.5599) (-18.422, -21.563) (-18.407, -21.566) (-18.3921, -21.5689) (-18.3771, -21.5718) (-18.3622, -21.5745) (-18.3473, -21.5773) (-18.3324, -21.5799) (-18.3175, -21.5825) (-18.3026, -21.5849) (-18.2877, -21.5874) (-18.2729, -21.5897) (-18.258, -21.5919) (-18.2432, -21.5941) (-18.2284, -21.5962) (-18.2136, -21.5983) (-18.1988, -21.6002) (-18.184, -21.6021) (-18.1693, -21.6039) (-18.1545, -21.6056) (-18.1398, -21.6072) (-18.1251, -21.6088) (-18.1104, -21.6102) (-18.0957, -21.6116) (-18.081, -21.6129) (-18.0664, -21.6141) (-18.0518, -21.6153) (-18.0372, -21.6163) (-18.0226, -21.6173) (-18.008, -21.6182) (-17.9935, -21.619) (-17.9789, -21.6197) (-17.9644, -21.6203) (-17.9499, -21.6208) (-17.9355, -21.6212) (-17.921, -21.6216) (-17.9066, -21.6218) (-17.8922, -21.622) (-17.8778, -21.622) (-17.8635, -21.622) (-17.8492, -21.6219) (-17.8349, -21.6217) (-17.8206, -21.6213) (-17.8064, -21.6209) (-17.7922, -21.6203) (-17.778, -21.6197) (-17.7638, -21.6189) (-17.7497, -21.618) (-17.7356, -21.617) (-17.7216, -21.6159) (-17.7076, -21.6147) (-17.6936, -21.6134) (-17.6796, -21.612) (-17.6657, -21.6103) (-17.6519, -21.6085) (-17.6381, -21.6066) (-17.6244, -21.6044) (-17.6107, -21.6022) (-17.597, -21.5998) (-17.5834, -21.5974) (-17.5698, -21.5949) (-17.5563, -21.5921) (-17.5429, -21.5889) (-17.5323, -21.586) (-17.5244, -21.5835) (-17.5192, -21.5818) (-17.5166, -21.5809) knots -1 -1 -1 -1 -1 -1 -0.98571429 -0.97142857 -0.95714286 -0.94285714 -0.92857143 -0.91428571 -0.9 -0.88571429 -0.87142857 -0.85714286 -0.84285714 -0.82857143 -0.81428571 -0.8 -0.78571429 -0.77142857 -0.75714286 -0.74285714 -0.72857143 -0.71428571 -0.7 -0.68571429 -0.67142857 -0.65714286 -0.64285714 -0.62857143 -0.61428571 -0.6 -0.58571429 -0.57142857 -0.55714286 -0.54285714 -0.52857143 -0.51428571 -0.5 -0.48571429 -0.47142857 -0.45714286 -0.44285714 -0.42857143 -0.41428571 -0.4 -0.38571429 -0.37142857 -0.35714286 -0.34285714 -0.32857143 -0.31428571 -0.3 -0.28571429 -0.27142857 -0.25714286 -0.24285714 -0.22857143 -0.21428571 -0.2 -0.18571429 -0.17142857 -0.15714286 -0.14285714 -0.12857143 -0.11428571 -0.1 -0.08571429 -0.07142857 -0.05714286 -0.04285714 -0.02857143 -0.01428571 0 0 0 0 0 0
  line L3 (-17.5166, -21.5809) -> (-17.452, -21.558)
  arc A7 (-17.1368, -21.7004) -> (-17.452, -21.558) centre (-17.3687, -21.7938) ccw
  arc A8 (-17.1368, -21.7004) -> (-17.0927, -21.8068) centre (-11.6741, -19.5) ccw
  arc A9 (-17.215, -22.1303) -> (-17.0927, -21.8068) centre (-17.3228, -21.9048) ccw
  line L4 (-17.215, -22.1303) -> (-17.2768, -22.1599)
  spline S4 degree 5 poles (-17.2768, -22.1599) (-17.2793, -22.161) (-17.2842, -22.1635) (-17.2915, -22.1673) (-17.301, -22.1727) (-17.3127, -22.18) (-17.3243, -22.1875) (-17.3357, -22.1953) (-17.347, -22.2033) (-17.3584, -22.2113) (-17.3696, -22.2194) (-17.3809, -22.2276) (-17.392, -22.236) (-17.4031, -22.2445) (-17.4141, -22.2531) (-17.4249, -22.262) (-17.4358, -22.2709) (-17.4465, -22.28) (-17.4572, -22.2892) (-17.4679, -22.2984) (-17.4785, -22.3078) (-17.489, -22.3173) (-17.4995, -22.3268) (-17.51, -22.3365) (-17.5204, -22.3462) (-17.5307, -22.3561) (-17.5409, -22.366) (-17.5512, -22.376) (-17.5613, -22.3862) (-17.5715, -22.3964) (-17.5815, -22.4067) (-17.5915, -22.417) (-17.6015, -22.4275) (-17.6114, -22.438) (-17.6213, -22.4486) (-17.6311, -22.4593) (-17.6409, -22.4701) (-17.6506, -22.481) (-17.6603, -22.4919) (-17.6699, -22.5029) (-17.6795, -22.5139) (-17.6891, -22.5251) (-17.6986, -22.5363) (-17.708, -22.5476) (-17.7174, -22.559) (-17.7268, -22.5704) (-17.7361, -22.5819) (-17.7453, -22.5935) (-17.7545, -22.6051) (-17.7637, -22.6168) (-17.7728, -22.6286) (-17.7819, -22.6404) (-17.7909, -22.6523) (-17.7999, -22.6643) (-17.8089, -22.6763) (-17.8178, -22.6884) (-17.8266, -22.7005) (-17.8354, -22.7128) (-17.8442, -22.725) (-17.8529, -22.7374) (-17.8616, -22.7498) (-17.8702, -22.7623) (-17.8788, -22.7748) (-17.8874, -22.7874) (-17.8959, -22.8) (-17.9043, -22.8127) (-17.9127, -22.8255) (-17.9211, -22.8383) (-17.9294, -22.8512) (-17.9377, -22.8641) (-17.9459, -22.8771) (-17.9525, -22.8875) (-17.9574, -22.8954) (-17.9606, -22.9006) (-17.9623, -22.9033) knots 0 0 0 0 0 0 0.01428571 0.02857143 0.04285714 0.05714286 0.07142857 0.08571429 0.1 0.11428571 0.12857143 0.14285714 0.15714286 0.17142857 0.18571429 0.2 0.21428571 0.22857143 0.24285714 0.25714286 0.27142857 0.28571429 0.3 0.31428571 0.32857143 0.34285714 0.35714286 0.37142857 0.38571429 0.4 0.41428571 0.42857143 0.44285714 0.45714286 0.47142857 0.48571429 0.5 0.51428571 0.52857143 0.54285714 0.55714286 0.57142857 0.58571429 0.6 0.61428571 0.62857143 0.64285714 0.65714286 0.67142857 0.68571429 0.7 0.71428571 0.72857143 0.74285714 0.75714286 0.77142857 0.78571429 0.8 0.81428571 0.82857143 0.84285714 0.85714286 0.87142857 0.88571429 0.9 0.91428571 0.92857143 0.94285714 0.95714286 0.97142857 0.98571429 1 1 1 1 1 1
  arc A10 (-17.9623, -22.9033) -> (-17.7655, -23.244) centre (-11.6741, -19.5) ccw
  spline S5 degree 5 poles (-17.7655, -23.244) (-17.7624, -23.2439) (-17.7562, -23.2438) (-17.747, -23.2434) (-17.7347, -23.243) (-17.7193, -23.2424) (-17.704, -23.2417) (-17.6887, -23.2409) (-17.6734, -23.24) (-17.6581, -23.2391) (-17.6429, -23.2382) (-17.6277, -23.2371) (-17.6125, -23.236) (-17.5974, -23.2349) (-17.5823, -23.2336) (-17.5672, -23.2323) (-17.5521, -23.2309) (-17.5371, -23.2295) (-17.5221, -23.228) (-17.5072, -23.2264) (-17.4923, -23.2247) (-17.4774, -23.223) (-17.4625, -23.2212) (-17.4477, -23.2193) (-17.4329, -23.2173) (-17.4181, -23.2153) (-17.4034, -23.2132) (-17.3887, -23.2111) (-17.3741, -23.2088) (-17.3595, -23.2065) (-17.3449, -23.2041) (-17.3304, -23.2017) (-17.3159, -23.1991) (-17.3014, -23.1965) (-17.287, -23.1938) (-17.2726, -23.1911) (-17.2583, -23.1882) (-17.244, -23.1853) (-17.2297, -23.1823) (-17.2155, -23.1792) (-17.2013, -23.1761) (-17.1872, -23.1728) (-17.1731, -23.1695) (-17.1591, -23.1661) (-17.1451, -23.1626) (-17.1311, -23.159) (-17.1172, -23.1554) (-17.1034, -23.1516) (-17.0896, -23.1478) (-17.0758, -23.1439) (-17.0621, -23.1399) (-17.0485, -23.1358) (-17.0349, -23.1315) (-17.0214, -23.1272) (-17.0079, -23.1228) (-16.9945, -23.1183) (-16.9812, -23.1137) (-16.9679, -23.109) (-16.9546, -23.1043) (-16.9415, -23.0994) (-16.9284, -23.0943) (-16.9154, -23.0892) (-16.9025, -23.0838) (-16.8897, -23.0784) (-16.877, -23.0728) (-16.8643, -23.067) (-16.8517, -23.0612) (-16.8391, -23.0554) (-16.8267, -23.0494) (-16.8144, -23.0432) (-16.8022, -23.0367) (-16.7928, -23.0311) (-16.7858, -23.0267) (-16.7812, -23.0237) (-16.779, -23.0221) knots -1 -1 -1 -1 -1 -1 -0.98571429 -0.97142857 -0.95714286 -0.94285714 -0.92857143 -0.91428571 -0.9 -0.88571429 -0.87142857 -0.85714286 -0.84285714 -0.82857143 -0.81428571 -0.8 -0.78571429 -0.77142857 -0.75714286 -0.74285714 -0.72857143 -0.71428571 -0.7 -0.68571429 -0.67142857 -0.65714286 -0.64285714 -0.62857143 -0.61428571 -0.6 -0.58571429 -0.57142857 -0.55714286 -0.54285714 -0.52857143 -0.51428571 -0.5 -0.48571429 -0.47142857 -0.45714286 -0.44285714 -0.42857143 -0.41428571 -0.4 -0.38571429 -0.37142857 -0.35714286 -0.34285714 -0.32857143 -0.31428571 -0.3 -0.28571429 -0.27142857 -0.25714286 -0.24285714 -0.22857143 -0.21428571 -0.2 -0.18571429 -0.17142857 -0.15714286 -0.14285714 -0.12857143 -0.11428571 -0.1 -0.08571429 -0.07142857 -0.05714286 -0.04285714 -0.02857143 -0.01428571 0 0 0 0 0 0
  line L5 (-16.779, -23.0221) -> (-16.7225, -22.9833)
  arc A11 (-16.3812, -23.0392) -> (-16.7225, -22.9833) centre (-16.581, -23.1895) ccw
  arc A12 (-16.3812, -23.0392) -> (-16.3111, -23.1307) centre (-11.6741, -19.5) ccw
  arc A13 (-16.3454, -23.4748) -> (-16.3111, -23.1307) centre (-16.5079, -23.2848) ccw
  line L6 (-16.3454, -23.4748) -> (-16.3975, -23.5193)
  spline S6 degree 5 poles (-16.3975, -23.5193) (-16.3995, -23.5211) (-16.4037, -23.5247) (-16.4097, -23.5303) (-16.4176, -23.538) (-16.427, -23.548) (-16.4362, -23.5583) (-16.4452, -23.5688) (-16.4541, -23.5794) (-16.4629, -23.5901) (-16.4717, -23.6008) (-16.4805, -23.6117) (-16.4891, -23.6226) (-16.4975, -23.6337) (-16.5059, -23.6449) (-16.5141, -23.6563) (-16.5223, -23.6677) (-16.5303, -23.6793) (-16.5383, -23.6909) (-16.5462, -23.7026) (-16.554, -23.7144) (-16.5617, -23.7263) (-16.5694, -23.7382) (-16.577, -23.7502) (-16.5845, -23.7623) (-16.5919, -23.7745) (-16.5993, -23.7868) (-16.6065, -23.7991) (-16.6137, -23.8115) (-16.6209, -23.824) (-16.6279, -23.8366) (-16.6349, -23.8492) (-16.6419, -23.8619) (-16.6487, -23.8746) (-16.6555, -23.8874) (-16.6622, -23.9003) (-16.6689, -23.9132) (-16.6755, -23.9262) (-16.682, -23.9393) (-16.6884, -23.9524) (-16.6948, -23.9656) (-16.7012, -23.9788) (-16.7074, -23.9921) (-16.7136, -24.0054) (-16.7198, -24.0188) (-16.7258, -24.0323) (-16.7319, -24.0458) (-16.7378, -24.0594) (-16.7437, -24.073) (-16.7495, -24.0867) (-16.7553, -24.1004) (-16.761, -24.1142) (-16.7666, -24.128) (-16.7722, -24.1419) (-16.7778, -24.1558) (-16.7832, -24.1698) (-16.7886, -24.1839) (-16.794, -24.198) (-16.7993, -24.2121) (-16.8045, -24.2263) (-16.8097, -24.2405) (-16.8148, -24.2548) (-16.8198, -24.2691) (-16.8248, -24.2834) (-16.8298, -24.2979) (-16.8346, -24.3123) (-16.8395, -24.3268) (-16.8442, -24.3414) (-16.8489, -24.356) (-16.8536, -24.3706) (-16.8582, -24.3853) (-16.8618, -24.3971) (-16.8645, -24.4059) (-16.8663, -24.4118) (-16.8672, -24.4148) knots 0 0 0 0 0 0 0.01428571 0.02857143 0.04285714 0.05714286 0.07142857 0.08571429 0.1 0.11428571 0.12857143 0.14285714 0.15714286 0.17142857 0.18571429 0.2 0.21428571 0.22857143 0.24285714 0.25714286 0.27142857 0.28571429 0.3 0.31428571 0.32857143 0.34285714 0.35714286 0.37142857 0.38571429 0.4 0.41428571 0.42857143 0.44285714 0.45714286 0.47142857 0.48571429 0.5 0.51428571 0.52857143 0.54285714 0.55714286 0.57142857 0.58571429 0.6 0.61428571 0.62857143 0.64285714 0.65714286 0.67142857 0.68571429 0.7 0.71428571 0.72857143 0.74285714 0.75714286 0.77142857 0.78571429 0.8 0.81428571 0.82857143 0.84285714 0.85714286 0.87142857 0.88571429 0.9 0.91428571 0.92857143 0.94285714 0.95714286 0.97142857 0.98571429 1 1 1 1 1 1
  arc A14 (-16.8672, -24.4148) -> (-16.5889, -24.693) centre (-11.6741, -19.5) ccw
  spline S7 degree 5 poles (-16.5889, -24.693) (-16.586, -24.6921) (-16.58, -24.6904) (-16.5712, -24.6877) (-16.5594, -24.684) (-16.5447, -24.6794) (-16.5301, -24.6748) (-16.5155, -24.6701) (-16.501, -24.6653) (-16.4865, -24.6605) (-16.472, -24.6556) (-16.4576, -24.6507) (-16.4432, -24.6457) (-16.4289, -24.6406) (-16.4146, -24.6355) (-16.4004, -24.6304) (-16.3862, -24.6251) (-16.3721, -24.6198) (-16.358, -24.6145) (-16.344, -24.6091) (-16.33, -24.6036) (-16.3161, -24.5981) (-16.3022, -24.5925) (-16.2883, -24.5869) (-16.2746, -24.5812) (-16.2608, -24.5754) (-16.2471, -24.5696) (-16.2335, -24.5637) (-16.22, -24.5577) (-16.2064, -24.5517) (-16.193, -24.5456) (-16.1796, -24.5395) (-16.1662, -24.5333) (-16.1529, -24.527) (-16.1397, -24.5207) (-16.1265, -24.5143) (-16.1134, -24.5078) (-16.1003, -24.5013) (-16.0873, -24.4947) (-16.0744, -24.4881) (-16.0615, -24.4814) (-16.0487, -24.4746) (-16.036, -24.4677) (-16.0233, -24.4608) (-16.0107, -24.4538) (-15.9982, -24.4467) (-15.9857, -24.4396) (-15.9733, -24.4324) (-15.9609, -24.4251) (-15.9487, -24.4178) (-15.9365, -24.4104) (-15.9244, -24.4029) (-15.9123, -24.3953) (-15.9004, -24.3876) (-15.8885, -24.3799) (-15.8768, -24.372) (-15.8651, -24.3641) (-15.8534, -24.3562) (-15.8419, -24.3481) (-15.8304, -24.34) (-15.8191, -24.3318) (-15.8078, -24.3234) (-15.7968, -24.3149) (-15.7858, -24.3063) (-15.775, -24.2976) (-15.7642, -24.2888) (-15.7536, -24.2799) (-15.743, -24.271) (-15.7325, -24.262) (-15.7222, -24.2529) (-15.7121, -24.2434) (-15.7044, -24.2356) (-15.6988, -24.2295) (-15.6952, -24.2254) (-15.6934, -24.2233) knots -1 -1 -1 -1 -1 -1 -0.98571429 -0.97142857 -0.95714286 -0.94285714 -0.92857143 -0.91428571 -0.9 -0.88571429 -0.87142857 -0.85714286 -0.84285714 -0.82857143 -0.81428571 -0.8 -0.78571429 -0.77142857 -0.75714286 -0.74285714 -0.72857143 -0.71428571 -0.7 -0.68571429 -0.67142857 -0.65714286 -0.64285714 -0.62857143 -0.61428571 -0.6 -0.58571429 -0.57142857 -0.55714286 -0.54285714 -0.52857143 -0.51428571 -0.5 -0.48571429 -0.47142857 -0.45714286 -0.44285714 -0.42857143 -0.41428571 -0.4 -0.38571429 -0.37142857 -0.35714286 -0.34285714 -0.32857143 -0.31428571 -0.3 -0.28571429 -0.27142857 -0.25714286 -0.24285714 -0.22857143 -0.21428571 -0.2 -0.18571429 -0.17142857 -0.15714286 -0.14285714 -0.12857143 -0.11428571 -0.1 -0.08571429 -0.07142857 -0.05714286 -0.04285714 -0.02857143 -0.01428571 0 0 0 0 0 0
  line L7 (-15.6934, -24.2233) -> (-15.6489, -24.1713)
  arc A15 (-15.3048, -24.1369) -> (-15.6489, -24.1713) centre (-15.4589, -24.3338) ccw
  arc A16 (-15.3048, -24.1369) -> (-15.2134, -24.2071) centre (-11.6741, -19.5) ccw
  arc A17 (-15.1575, -24.5484) -> (-15.2134, -24.2071) centre (-15.3636, -24.4069) ccw
  line L8 (-15.1575, -24.5484) -> (-15.1962, -24.6048)
  spline S8 degree 5 poles (-15.1962, -24.6048) (-15.1978, -24.6071) (-15.2009, -24.6117) (-15.2053, -24.6186) (-15.2108, -24.6281) (-15.2173, -24.6402) (-15.2235, -24.6525) (-15.2295, -24.665) (-15.2354, -24.6776) (-15.2412, -24.6902) (-15.2469, -24.7028) (-15.2525, -24.7155) (-15.258, -24.7283) (-15.2633, -24.7412) (-15.2685, -24.7542) (-15.2735, -24.7673) (-15.2784, -24.7805) (-15.2832, -24.7937) (-15.2879, -24.807) (-15.2924, -24.8204) (-15.297, -24.8338) (-15.3014, -24.8473) (-15.3057, -24.8608) (-15.3099, -24.8744) (-15.314, -24.888) (-15.318, -24.9017) (-15.3219, -24.9154) (-15.3258, -24.9292) (-15.3295, -24.9431) (-15.3332, -24.957) (-15.3368, -24.9709) (-15.3402, -24.9849) (-15.3437, -24.999) (-15.347, -25.013) (-15.3502, -25.0272) (-15.3534, -25.0413) (-15.3565, -25.0556) (-15.3595, -25.0698) (-15.3624, -25.0841) (-15.3652, -25.0985) (-15.368, -25.1128) (-15.3707, -25.1273) (-15.3733, -25.1417) (-15.3758, -25.1562) (-15.3783, -25.1708) (-15.3807, -25.1853) (-15.383, -25.2) (-15.3852, -25.2146) (-15.3874, -25.2293) (-15.3895, -25.244) (-15.3915, -25.2588) (-15.3934, -25.2735) (-15.3953, -25.2884) (-15.3971, -25.3032) (-15.3988, -25.3181) (-15.4005, -25.333) (-15.4021, -25.348) (-15.4036, -25.363) (-15.4051, -25.378) (-15.4064, -25.3931) (-15.4078, -25.4081) (-15.409, -25.4232) (-15.4102, -25.4384) (-15.4113, -25.4536) (-15.4123, -25.4688) (-15.4133, -25.484) (-15.4142, -25.4992) (-15.415, -25.5145) (-15.4158, -25.5298) (-15.4165, -25.5452) (-15.4171, -25.5605) (-15.4176, -25.5729) (-15.4179, -25.5821) (-15.4181, -25.5883) (-15.4182, -25.5914) knots 0 0 0 0 0 0 0.01428571 0.02857143 0.04285714 0.05714286 0.07142857 0.08571429 0.1 0.11428571 0.12857143 0.14285714 0.15714286 0.17142857 0.18571429 0.2 0.21428571 0.22857143 0.24285714 0.25714286 0.27142857 0.28571429 0.3 0.31428571 0.32857143 0.34285714 0.35714286 0.37142857 0.38571429 0.4 0.41428571 0.42857143 0.44285714 0.45714286 0.47142857 0.48571429 0.5 0.51428571 0.52857143 0.54285714 0.55714286 0.57142857 0.58571429 0.6 0.61428571 0.62857143 0.64285714 0.65714286 0.67142857 0.68571429 0.7 0.71428571 0.72857143 0.74285714 0.75714286 0.77142857 0.78571429 0.8 0.81428571 0.82857143 0.84285714 0.85714286 0.87142857 0.88571429 0.9 0.91428571 0.92857143 0.94285714 0.95714286 0.97142857 0.98571429 1 1 1 1 1 1
  arc A18 (-15.4182, -25.5914) -> (-15.0774, -25.7881) centre (-11.6741, -19.5) ccw
  spline S9 degree 5 poles (-15.0774, -25.7881) (-15.0748, -25.7865) (-15.0695, -25.7832) (-15.0617, -25.7783) (-15.0512, -25.7718) (-15.0382, -25.7636) (-15.0253, -25.7553) (-15.0124, -25.747) (-14.9996, -25.7386) (-14.9868, -25.7302) (-14.9741, -25.7217) (-14.9615, -25.7132) (-14.9489, -25.7047) (-14.9364, -25.6961) (-14.9239, -25.6875) (-14.9115, -25.6788) (-14.8992, -25.6701) (-14.8869, -25.6613) (-14.8747, -25.6525) (-14.8625, -25.6436) (-14.8504, -25.6347) (-14.8384, -25.6258) (-14.8264, -25.6168) (-14.8145, -25.6078) (-14.8027, -25.5987) (-14.7909, -25.5896) (-14.7792, -25.5804) (-14.7676, -25.5712) (-14.756, -25.5619) (-14.7445, -25.5526) (-14.7331, -25.5433) (-14.7217, -25.5339) (-14.7104, -25.5244) (-14.6992, -25.5149) (-14.6881, -25.5054) (-14.677, -25.4958) (-14.666, -25.4862) (-14.6551, -25.4765) (-14.6442, -25.4668) (-14.6335, -25.457) (-14.6228, -25.4472) (-14.6122, -25.4373) (-14.6016, -25.4274) (-14.5912, -25.4174) (-14.5808, -25.4074) (-14.5705, -25.3973) (-14.5603, -25.3872) (-14.5502, -25.377) (-14.5402, -25.3668) (-14.5302, -25.3565) (-14.5204, -25.3462) (-14.5106, -25.3358) (-14.5009, -25.3254) (-14.4914, -25.3149) (-14.4819, -25.3044) (-14.4726, -25.2937) (-14.4633, -25.2831) (-14.4541, -25.2724) (-14.4451, -25.2616) (-14.4361, -25.2508) (-14.4273, -25.2399) (-14.4186, -25.2289) (-14.4101, -25.2179) (-14.4017, -25.2067) (-14.3935, -25.1955) (-14.3854, -25.1842) (-14.3774, -25.1729) (-14.3695, -25.1616) (-14.3617, -25.1501) (-14.3541, -25.1386) (-14.3469, -25.1269) (-14.3414, -25.1174) (-14.3376, -25.1101) (-14.3352, -25.1051) (-14.334, -25.1026) knots -1 -1 -1 -1 -1 -1 -0.98571429 -0.97142857 -0.95714286 -0.94285714 -0.92857143 -0.91428571 -0.9 -0.88571429 -0.87142857 -0.85714286 -0.84285714 -0.82857143 -0.81428571 -0.8 -0.78571429 -0.77142857 -0.75714286 -0.74285714 -0.72857143 -0.71428571 -0.7 -0.68571429 -0.67142857 -0.65714286 -0.64285714 -0.62857143 -0.61428571 -0.6 -0.58571429 -0.57142857 -0.55714286 -0.54285714 -0.52857143 -0.51428571 -0.5 -0.48571429 -0.47142857 -0.45714286 -0.44285714 -0.42857143 -0.41428571 -0.4 -0.38571429 -0.37142857 -0.35714286 -0.34285714 -0.32857143 -0.31428571 -0.3 -0.28571429 -0.27142857 -0.25714286 -0.24285714 -0.22857143 -0.21428571 -0.2 -0.18571429 -0.17142857 -0.15714286 -0.14285714 -0.12857143 -0.11428571 -0.1 -0.08571429 -0.07142857 -0.05714286 -0.04285714 -0.02857143 -0.01428571 0 0 0 0 0 0
  line L9 (-14.334, -25.1026) -> (-14.3045, -25.0408)
  arc A19 (-13.981, -24.9186) -> (-14.3045, -25.0408) centre (-14.0789, -25.1486) ccw
  arc A20 (-13.981, -24.9186) -> (-13.8745, -24.9627) centre (-11.6741, -19.5) ccw
  arc A21 (-13.7322, -25.2779) -> (-13.8745, -24.9627) centre (-13.9679, -25.1946) ccw
  line L10 (-13.7322, -25.2779) -> (-13.755, -25.3425)